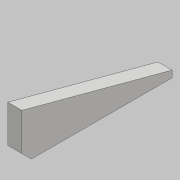
# Autodesk Inventor part: exercise3-18
Saved by Autodesk Inventor 2018 (Build 220112000, 112)
## iProperties
Created: 2020-09-23
Part Number: exercise3-18
Material: 一般
Document SubType Name: Modeling
Designer: 王鼎鈞
Density: 1 g/cm^3
Appearance: 預設
Author: 王鼎鈞
Autodesk Inventor part; units mm, degrees
ref_plane "YZ Plane" through (0, 0, 0) normal (1, 0, 0) x (0, 1, 0)
ref_plane "XZ Plane" through (0, 0, 0) normal (0, 1, 0) x (-1, 0, 0)
ref_plane "XY Plane" through (0, 0, 0) normal (0, 0, 1) x (1, 0, 0)
sketch "草圖1" plane through (0, 0, 0) normal (1, 0, 0) x (0, 1, 0)
  line L0 (-32, 0) -> (192, 0) projected
  line L1 (0, -10) -> (0, 60) projected
  line L2 (0, 0) -> (160, 0)
  line L3 (160, 0) -> (160, 50)
  line L4 (160, 50) -> (0, 50)
  line L5 (0, 50) -> (0, 0)
  line L6 (0, 50) -> (160, 7.1281)
  dimension "d0" = 160
  dimension "d1" = 50
  dimension "d2" = 75
  constraints: 10 end point, 2 parallel, 1 horizontal, 1 perpendicular, 1 point on line
  measures "d0" distance of L4.end L3.end
  measures "d1" distance of L3.end L2.end
  measures "d2" angle of L5 L6
extrude "擠出1" add sketch "草圖1" along normal blind 15 contours L1 L6 L3 L0
chamfer "倒角1" distance 10 angle 45 1 edges at (7.5, 0, 0)
